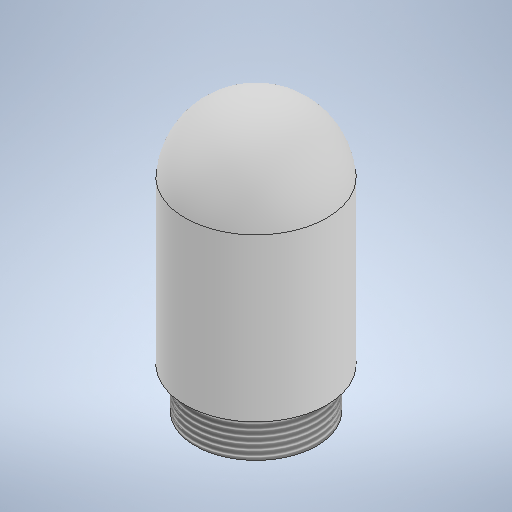
# Autodesk Inventor part: bulb
Saved by Autodesk Inventor 2025.2 (Build 292293000, 293)
## iProperties
Created: 2025-09-04
Part Number: bulb
Material: Generic
Document SubType Name: Modeling
Designer: User
Density: 1 g/cm^3
Appearance: Default
Author: User
Autodesk Inventor part; units mm, degrees
ref_plane "YZ Plane" through (0, 0, 0) normal (1, 0, 0) x (0, 1, 0)
ref_plane "XZ Plane" through (0, 0, 0) normal (0, 1, 0) x (-1, 0, 0)
ref_plane "XY Plane" through (0, 0, 0) normal (0, 0, 1) x (1, 0, 0)
sketch "Sketch1" plane through (0, 0, 0) normal (0, 0, 1) x (1, 0, 0)
  point P0 (0, 0)
sketch "Sketch2" plane through (0, 0, 0) normal (0, 0, 1) x (1, 0, 0)
  line L0 (0, 0) -> (0, 142.875)
  line L1 (0, 0) -> (44.45, 0)
  line L2 (44.45, 0) -> (44.45, 101.6)
  arc A0 (44.45, 101.6) -> (0, 142.875) centre (0.3432, 98.6724) ccw
  dimension "d0" = 101.6
  dimension "d1" = 142.875
  dimension "d2" = 44.45
  constraints: 6 end point, 2 point on circle, 1 centre point, 1 horizontal, 1 perpendicular, 1 vertical
  measures "d0" distance from line of L2.end L1
  measures "d1" distance of L0.start L0.end
  measures "d2" distance between parallel lines of L0 L2
revolve "Revolution1" add sketch "Sketch2" angle 360 about axis through (0, 0, 0) along (0, 1, 0)
sketch "Sketch3" plane through (0, 0, 0) normal (0, -1, 0) x (1, 0, 0)
  circle A0 centre (0, 0) radius 38.1
  dimension "d4" = 76.2
  constraints: 1 centre point, 1 coincident
  measures "d4" diameter of A0
extrude "Extrusion1" add sketch "Sketch3" along normal blind 25.4
thread "Thread1" size "1 1/8-7 UNC" class "2A" standard "ANSI Unified Screw Threads" full length
body "Solid1"
